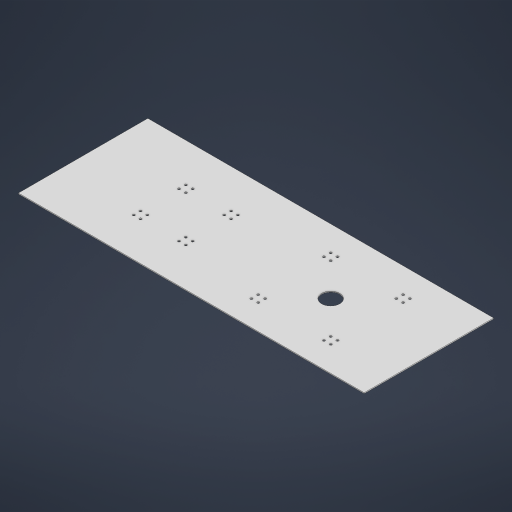
# Autodesk Inventor part: ChassisTop
Saved by Autodesk Inventor 2024 (Build 280153000, 153)
## iProperties
Created: 2023-10-19
Part Number: ChassisTop
Material: Generic
Document SubType Name: Modeling
Designer: avsar
Density: 1 g/cm^3
Appearance: Default
Author: avsar
Autodesk Inventor part; units mm, degrees
ref_plane "YZ Plane" through (0, 0, 0) normal (1, 0, 0) x (0, 1, 0)
ref_plane "XZ Plane" through (0, 0, 0) normal (0, 1, 0) x (-1, 0, 0)
ref_plane "XY Plane" through (0, 0, 0) normal (0, 0, 1) x (1, 0, 0)
sketch "Sketch1" plane through (0, 0, 0) normal (0, 1, 0) x (-1, 0, 0)
  line L0 (305.435, 114.3) -> (-305.435, 114.3)
  line L1 (-305.435, 114.3) -> (-305.435, -114.3)
  line L2 (-305.435, -114.3) -> (305.435, -114.3)
  line L3 (305.435, -114.3) -> (305.435, 114.3)
  line L4 (305.435, 114.3) -> (-305.435, -114.3) construction
  line L5 (-305.435, 114.3) -> (305.435, -114.3) construction
  point P0 (0, 0)
  dimension "d0" = 610.87
  dimension "d1" = 228.6
  constraints: 12 end point, 2 midpoint, 2 parallel, 1 horizontal, 1 perpendicular
  measures "d0" distance of L2.end L1.end
  measures "d1" distance of L1.end L0.end
extrude "Extrusion1" add sketch "Sketch1" along normal mid plane 1.5875
sketch "Sketch2" plane through (0, 0.7937, 0) normal (0, 1, 0) x (1, 0, 0)
  circle A0 centre (132, 0) radius 16
  circle A1 centre (196, -64) radius 2.5 construction
  circle A2 centre (202, -70) radius 2
  circle A3 centre (202, -58) radius 2
  circle A4 centre (190, -58) radius 2
  circle A5 centre (190, -70) radius 2
  circle A6 centre (190, 58) radius 2
  circle A7 centre (202, 58) radius 2
  circle A8 centre (202, 70) radius 2
  circle A9 centre (190, 70) radius 2
  circle A10 centre (74, 58) radius 2
  circle A11 centre (74, 70) radius 2
  circle A12 centre (62, 70) radius 2
  circle A13 centre (62, 58) radius 2
  circle A14 centre (74, -58) radius 2
  circle A15 centre (62, -58) radius 2
  circle A16 centre (62, -70) radius 2
  circle A17 centre (74, -70) radius 2
  point P0 (0, 0)
  dimension "d4" = 32
  dimension "d5" = 132
  dimension "d6" = 5
  dimension "d7" = 64
  dimension "d8" = 64
  dimension "d11" = 4
  dimension "d12" = 6
  dimension "d13" = 6
  dimension "d16" = 360
  dimension "d20" = 360
  constraints: 18 centre point, 1 horizontal alignment, 42 other
  measures "d4" diameter of A0
  measures "d5" distance of A0.centre point (0, 0)
  measures "d6" diameter of A1
  measures "d7" horizontal distance of A1.centre A0.centre
  measures "d8" horizontal distance of A1.centre A0.centre
  measures "d11" diameter of A2
  measures "d12" horizontal distance of A1.centre A2.centre
  measures "d13" horizontal distance of A2.centre A1.centre
extrude "Extrusion2" cut sketch "Sketch2" against normal through all
sketch "Sketch3" plane through (0, 0.7937, 0) normal (0, 1, 0) x (1, 0, 0)
  circle A0 centre (-124, 0) radius 7 construction
  circle A1 centre (132, 0) radius 16 construction
  circle A2 centre (-164, -40) radius 2.5 construction
  circle A3 centre (-158, -34) radius 2
  circle A4 centre (-170, -34) radius 2
  circle A5 centre (-170, -46) radius 2
  circle A6 centre (-158, -46) radius 2
  circle A7 centre (-90, -46) radius 2
  circle A8 centre (-90, -34) radius 2
  circle A9 centre (-78, -46) radius 2
  circle A10 centre (-78, -34) radius 2
  circle A11 centre (-78, 34) radius 2
  circle A12 centre (-90, 34) radius 2
  circle A13 centre (-78, 46) radius 2
  circle A14 centre (-90, 46) radius 2
  circle A15 centre (-158, 46) radius 2
  circle A16 centre (-158, 34) radius 2
  circle A17 centre (-170, 46) radius 2
  circle A18 centre (-170, 34) radius 2
  point P0 (0, 0)
  dimension "d24" = 14
  dimension "d25" = 256
  dimension "d42" = 5
  dimension "d43" = 40
  dimension "d44" = 40
  dimension "d45" = 4
  dimension "d46" = 6
  dimension "d47" = 6
  dimension "d50" = 360
  dimension "d54" = 360
  constraints: 18 centre point, 1 horizontal alignment, 42 other
  measures "d24" diameter of A0
  measures "d25" distance of A1.centre A0.centre
  measures "d42" diameter of A2
  measures "d43" horizontal distance of A0.centre A2.centre
  measures "d44" horizontal distance of A0.centre A2.centre
  measures "d45" diameter of A3
  measures "d46" horizontal distance of A3.centre A2.centre
  measures "d47" horizontal distance of A2.centre A3.centre
extrude "Extrusion4" cut sketch "Sketch3" against normal through all
body "Solid1"
